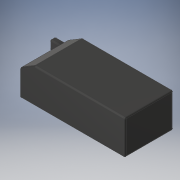
# Autodesk Inventor part: Akku
Saved by Autodesk Inventor 2018 (Build 220112000, 112)
## iProperties
Created: 2019-03-04
Part Number: Akku
Material: Aluminium 6061
Document SubType Name: Modeling
Designer: RedBots
Density: 2.00784 g/cm^3
Appearance: Glatt - schwarz
Mass: 130 g
Surface Area: 105.244 cm^2
Volume: 64.7462 cm^3
Author: RedBots
Autodesk Inventor part; units mm, degrees
ref_plane "YZ Plane" through (0, 0, 0) normal (1, 0, 0) x (0, 1, 0)
ref_plane "XZ Plane" through (0, 0, 0) normal (0, 1, 0) x (-1, 0, 0)
ref_plane "XY Plane" through (0, 0, 0) normal (0, 0, 1) x (1, 0, 0)
sketch "Skizze1" plane through (0, 0, 0) normal (0, 0, 1) x (1, 0, 0)
  line L0 (0, 0) -> (75, 0)
  line L1 (75, 0) -> (75, 35)
  line L2 (75, 35) -> (0, 35)
  line L3 (0, 35) -> (0, 0)
  dimension "d0" = 75
  dimension "d1" = 35
  constraints: 8 end point, 2 parallel, 1 horizontal, 1 perpendicular
  measures "d0" distance of L2.end L1.end
  measures "d1" distance of L1.end L0.end
extrude "Extrusion1" add sketch "Skizze1" along normal blind 25
sketch "Skizze3" plane through (0, 0, 0) normal (0, -1, 0) x (1, 0, 0)
  line L0 (0, 25) -> (75, 25) projected
  line L1 (0, 25) -> (0, 19)
  line L2 (0, 0) -> (0, 25) projected
  line L3 (0, 19) -> (10, 25)
  line L4 (10, 25) -> (0, 25)
  point P0 (74, 25)
  dimension "d9" = 6
  dimension "d10" = 10
  constraints: 6 end point, 1 perpendicular, 1 point on line
  measures "d9" distance of L0.start L1.end
  measures "d10" distance of L3.end L0.start
extrude "Extrusion3" cut sketch "Skizze3" against normal up to next
fillet "Rundung2" radius 1 13 edges at (10, 17.5, 25) (42.5, 0, 25) (42.5, 35, 25) (75, 17.5, 25) (75, 35, 12.5) (75, 0, 12.5) (75, 17.5, 0) (37.5, 0, 0) (5, 0, 22) (0, 17.5, 0) (0, 17.5, 19) (37.5, 35, 0) (5, 35, 22)
sketch "Skizze5" plane through (0, 0, 1) normal (-1, 0, 0) x (0, 0, 1)
  line L0 (0, 35) -> (23, 35) projected
  line L1 (8, 35) -> (15, 35)
  line L2 (15, 35) -> (15, 31)
  line L3 (15, 31) -> (8, 31)
  line L4 (8, 31) -> (8, 35)
  point P0 (-1, 0)
  point P1 (11.5, 35)
  dimension "d14" = 7
  dimension "d15" = 4
  constraints: 8 end point, 2 midpoint, 2 parallel, 1 horizontal, 1 perpendicular, 1 point on line
  measures "d14" distance of L2.end L3.end
  measures "d15" distance of L1.end L2.end
extrude "Extrusion4" add sketch "Skizze5" along normal blind 10
fillet "Rundung3" radius 1 11 edges at (0, 31, 12.5) (0, 33, 16) (0, 33, 9) (-5, 31, 9) (-10, 33, 9) (-10, 31, 12.5) (-10, 33, 16) (-5, 31, 16) (-5, 35, 16) (-5, 35, 9) (-10, 35, 12.5)
